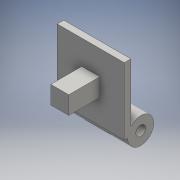
# Autodesk Inventor part: camera holder
Saved by Autodesk Inventor 2016 (Build 200138000, 138)
## iProperties
Created: 2015-10-02
Part Number: camera holder
Material: Generic
Document SubType Name: Modeling
Designer: Zachary
Density: 1 g/cm^3
Appearance: Default
Author: Zachary
Autodesk Inventor part; units mm, degrees
ref_plane "YZ Plane" through (0, 0, 0) normal (1, 0, 0) x (0, 1, 0)
ref_plane "XZ Plane" through (0, 0, 0) normal (0, 1, 0) x (-1, 0, 0)
ref_plane "XY Plane" through (0, 0, 0) normal (0, 0, 1) x (1, 0, 0)
sketch "Sketch1" plane through (0, 0, 0) normal (0, 1, 0) x (-1, 0, 0)
  line L0 (0, 0) -> (5.5, 0)
  line L1 (5.5, 0) -> (5.5, -5.5)
  line L2 (5.5, -5.5) -> (0, -5.5)
  line L3 (0, -5.5) -> (0, 0)
  dimension "d0" = 5.5
  dimension "d1" = 5.5
  constraints: 8 end point, 2 parallel, 1 horizontal, 1 perpendicular
  measures "d0" distance of L1.end L2.end
  measures "d1" distance of L0.end L1.end
extrude "Extrusion1" add sketch "Sketch1" along normal blind 9.5
sketch "Sketch2" plane through (0, 9.5, 0) normal (0, 1, 0) x (1, 0, 0)
  line L0 (-5.5, 5.5) -> (-5.5, 0) projected
  line L1 (-5.5, 2.75) -> (0, 2.75)
  line L2 (-2.75, 5.5) -> (-2.75, 0)
  line L3 (7.5, -7.5) -> (-13, -7.5)
  line L4 (-13, -7.5) -> (-13, 13)
  line L5 (-13, 13) -> (7.5, 13)
  line L6 (7.5, 13) -> (7.5, -7.5)
  line L7 (7.5, -7.5) -> (-13, 13) construction
  line L8 (-13, -7.5) -> (7.5, 13) construction
  point P0 (0, 0)
  point P1 (-2.75, 2.75)
  dimension "d4" = 20.5
  dimension "d5" = 20.5
  constraints: 16 end point, 4 midpoint, 2 horizontal, 2 parallel, 1 perpendicular, 1 vertical
  measures "d4" distance of L4.end L5.end
  measures "d5" distance of L3.end L4.end
extrude "Extrusion2" add sketch "Sketch2" along normal blind 2
sketch "Sketch4" plane through (7.5, 9.5, 7.5) normal (1, 0, 0) x (0, 0, -1)
  line L0 (0, 2) -> (20.5, 2) projected
  line L1 (20.5, 2) -> (20.5, 5)
  circle A0 centre (20.5, 5) radius 4
  point P0 (7.5, -9.5)
  dimension "d8" = 3
  constraints: 2 end point, 1 centre point, 1 coincident, 1 vertical
  measures "d8" distance of L0.end L1.end
extrude "Extrusion3" add sketch "Sketch4" against normal blind 20.5
hole "Hole1" at (-13, 14.5, -13) direction (1, 0, 0) diameter 3 end through all
sketch "Sketch5" plane through (-13, 9.5, 7.5) normal (0, 0, 1) x (1, 0, 0)
  line L0 (0, 2) -> (20.5, 2) projected
  line L1 (6.5, 2) -> (14, 2)
  line L2 (14, 2) -> (14, 14.1899)
  line L3 (14, 14.1899) -> (6.5, 14.1899)
  line L4 (6.5, 14.1899) -> (6.5, 2)
  line L5 (0, 9) -> (0, 1) projected
  line L6 (20.5, 9) -> (20.5, 1) projected
  point P0 (13, -9.5)
  dimension "d20" = 12.1899
  dimension "d21" = 6.5
  dimension "d22" = 6.5
  dimension "d23" = 7.5
  constraints: 8 end point, 2 parallel, 1 horizontal, 1 perpendicular, 1 point on line
  measures "d20" distance of L3.end L1.start
  measures "d21" distance between parallel lines of L4 L5
  measures "d22" distance between parallel lines of L6 L2
  measures "d23" distance of L2.end L3.end
extrude "Extrusion4" cut sketch "Sketch5" against normal blind 30
body "Solid1"
